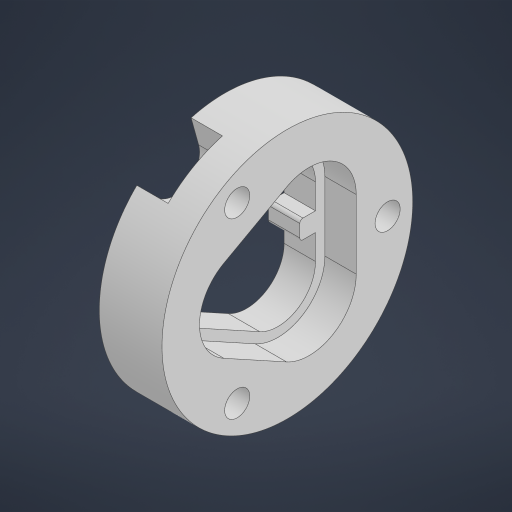
# Autodesk Inventor part: cap
Saved by Autodesk Inventor 2024 (Build 280153000, 153)
## iProperties
Created: 2024-06-02
Part Number: cap
Material: Generic
Document SubType Name: Modeling
Designer: markm
Density: 1 g/cm^3
Appearance: Default
Author: markm
Autodesk Inventor part; units mm, degrees
ref_plane "YZ Plane" through (0, 0, 0) normal (1, 0, 0) x (0, 1, 0)
ref_plane "XZ Plane" through (0, 0, 0) normal (0, 1, 0) x (-1, 0, 0)
ref_plane "XY Plane" through (0, 0, 0) normal (0, 0, 1) x (1, 0, 0)
sketch "Sketch1" plane through (0, 0, 0) normal (1, 0, 0) x (0, 1, 0)
  line L0 (-2.75, -5.2438) -> (2.75, -5.2438)
  line L1 (5.8168, -0.057) -> (3.0668, 4.943)
  line L2 (-3.0668, 4.943) -> (-5.8168, -0.057)
  line L3 (0, -5.2438) -> (0, 0) construction
  line L4 (0, 0) -> (-4.4418, 2.443) construction
  line L5 (0, 0) -> (4.4418, 2.443) construction
  arc A0 (-5.8168, -0.057) -> (-2.75, -5.2438) centre (-2.75, -1.7438) ccw
  arc A1 (3.0668, 4.943) -> (-3.0668, 4.943) centre (0, 3.2563) ccw
  arc A2 (2.75, -5.2438) -> (5.8168, -0.057) centre (2.75, -1.7438) ccw
  circle A3 centre (0, 0) radius 10
  circle A4 centre (0, -8) radius 2
  circle A5 centre (0, -8) radius 1
  line L6 (-2.75, -4.2438) -> (2.75, -4.2438)
  arc A6 (2.75, -4.2438) -> (4.9405, -0.539) centre (2.75, -1.7438) ccw
  line L7 (4.9405, -0.539) -> (2.1905, 4.461)
  arc A7 (2.1905, 4.461) -> (-2.1905, 4.461) centre (0, 3.2563) ccw
  line L8 (-2.1905, 4.461) -> (-4.9405, -0.539)
  arc A8 (-4.9405, -0.539) -> (-2.75, -4.2438) centre (-2.75, -1.7438) ccw
  line L9 (-1, -4.2438) -> (-1, -3.7438)
  line L10 (-0.5, -3.2438) -> (0.5, -3.2438)
  line L11 (1, -3.7438) -> (1, -4.2438)
  arc A9 (-0.5, -3.2438) -> (-1, -3.7438) centre (-0.5, -3.7438) ccw
  arc A10 (1, -3.7438) -> (0.5, -3.2438) centre (0.5, -3.7438) ccw
  line L12 (-33.0688, -12.3722) -> (-33.0688, 1.7139) construction
  line L13 (-33.0688, 1.7139) -> (-18.9827, 1.7139) construction
  line L14 (-18.9827, 1.7139) -> (-18.9827, -12.3722) construction
  line L15 (-18.9827, -12.3722) -> (-33.0688, -12.3722) construction
  line L16 (1.9365, -7.5) -> (2.5, -9.6825)
  line L17 (-1.9365, -7.5) -> (-2.5, -9.6825)
  point P0 (0, 6.7563)
  point P1 (-1, -3.2438)
  point P2 (0, -10)
  dimension "d0" = 3.5
  dimension "d1" = 20
  dimension "d3" = 4
  dimension "d4" = 2
  dimension "d9" = 12
  dimension "d10" = 12.5
  dimension "d11" = 5.5
  dimension "d12" = 1
  dimension "d24" = 2
  dimension "d25" = 1
  dimension "d26" = 0.5
  constraints: 28 end point, 21 point on circle, 13 tangent, 11 centre point, 5 point on line, 3 coincident, 3 equal radius, 3 midpoint, 3 perpendicular, 2 line through centre, 1 equal length, 1 horizontal, 9 other
  measures "d0" radius of A0
  measures "d1" diameter of A3
  measures "d3" diameter of A4
  measures "d4" diameter of A5
  measures "d9" distance from line of point (0, 6.756) L0
  measures "d11" distance of A2.centre A0.centre
  measures "d12" radial gap between concentric circles of A0 A8
  measures "d24" distance between parallel lines of L11 L9
  measures "d25" distance of L9.start point (-1, -3.244)
  measures "d26" radius of A9
extrude "Extrusion1" add sketch "Sketch1" against normal blind 2.5 contours A0 L2 A1 L1 A2 L0 | A3 L16 A4 L17 | L17 A4 A3 | A3 A4 L16 | A4 | A5 | L9 A9 L10 A10 L11 L6
extrude "Extrusion2" add sketch "Sketch1" along normal blind 2.5 contours A3 L16 A4 L17 | L17 A4 A3 | A3 A4 L16 | A4 | A5
extrude "Extrusion4" cut sketch "Sketch1" against normal through all contours L17 A4 A3 | A3 A4 L16 | A4
extrude "Extrusion3" cut sketch "Sketch1" along normal through all both and the other way through all contours A5
pattern_circular "Circular Pattern1" count 3 over 360 about axis through (0, 0, 0) along (-1, 0, 0) of "Extrusion4", "Extrusion3"
thicken "Thicken1" operation add thickness 0.5 both sides no extend neighbours yes toward (0, 0, -1) faces at (-0.8333, 2.1667, -4.2438) (-1.6667, 4.4868, -3.542) (-0.8333, -1.5833, -4.2438) (-1.6667, -5.0265, -0.7106) (-0.8333, 3.1072, 2.7944) (-1.6667, -1.5572, 5.212) (-1.6667, -4.0239, 1.1277)
thicken "Thicken2" operation add thickness 0.25 both sides no extend neighbours yes toward (0, -1, 0) faces at (-0.8333, 1, -4.4104) (-1.6667, 0.8401, -3.3772) (-0.8333, 0.1667, -3.2438) (-1.6667, -0.933, -3.4938) (-0.8333, -1, -4.0771) (0.8333, 0.9167, -5.2438) (1.6667, 3.8084, -5.0799) (1.6667, -5.3675, -4.0673) (0.8333, -4.9001, 1.6096) (1.6667, -0.6877, 6.688) (0.8333, 3.9834, 3.2763)
body "Solid1"
